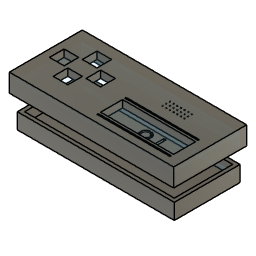
HardwareExam_LaurensController (Autodesk Fusion 360 design; units mm, degrees)
Autodesk Fusion 360 part; units mm, degrees
sketch "Sketch1" plane through (0, 0, 0) normal (0, 0, 1) x (1, 0, 0)
  line L0 (0, 110) -> (450, 110)
  line L1 (450, 110) -> (450, -90)
  line L2 (450, -90) -> (0, -90)
  line L3 (0, -90) -> (0, 110)
  dimension "d1" = 450
  dimension "d2" = 200
  constraint horizontal L0
  constraint vertical L1
  constraint horizontal L2
  constraint vertical L3
  measures "d1" distance of L0.start L0.end
  measures "d2" distance of L0.start L2.end
extrude "Extrude1" add sketch "Sketch1" against normal blind 30 makes body 1
sketch "Sketch2" plane through (0, 0, 0) normal (0, 0, 1) x (-1, 0, 0)
  line L0 (0, 90) -> (-450, 90)
  line L1 (-450, 90) -> (-450, -110)
  line L2 (-450, -110) -> (0, -110)
  line L3 (0, -110) -> (0, 90)
  line L4 (-220, 0) -> (-420, 0)
  line L5 (-420, 0) -> (-420, 60)
  line L6 (-420, 60) -> (-220, 60)
  line L7 (-220, 60) -> (-220, 0)
  line L8 (-70, -80) -> (-110, -80)
  line L9 (-110, -80) -> (-110, -40)
  line L10 (-110, -40) -> (-70, -40)
  line L11 (-70, -40) -> (-70, -80)
  line L12 (-110, 0) -> (-110, 40)
  line L13 (-70, 0) -> (-110, 0)
  line L14 (-70, 40) -> (-70, 0)
  line L15 (-110, 40) -> (-70, 40)
  line L16 (-160, -40) -> (-160, 0)
  line L17 (-120, -40) -> (-160, -40)
  line L18 (-120, 0) -> (-120, -40)
  line L19 (-160, 0) -> (-120, 0)
  line L20 (-60, -40) -> (-60, 0)
  line L21 (-20, -40) -> (-60, -40)
  line L22 (-20, 0) -> (-20, -40)
  line L23 (-60, 0) -> (-20, 0)
  dimension "d5" = 200
  dimension "d6" = 40
  dimension "d7" = 40
  dimension "d8" = 40
  dimension "d9" = 40
  dimension "d10" = 40
  dimension "d11" = 40
  dimension "d12" = 40
  dimension "d13" = 40
  constraint horizontal L4
  constraint vertical L5
  constraint horizontal L6
  constraint vertical L7
  constraint horizontal L8
  constraint vertical L9
  constraint horizontal L10
  constraint vertical L11
  constraint horizontal L13
  constraint vertical L12
  constraint horizontal L15
  constraint vertical L14
  constraint horizontal L17
  constraint vertical L16
  constraint horizontal L19
  constraint vertical L18
  constraint horizontal L21
  constraint vertical L20
  constraint horizontal L23
  constraint vertical L22
  measures "d5" distance of L4.start L4.end
  measures "d6" distance of L8.start L8.end
  measures "d7" distance of L8.start L10.end
  measures "d8" distance of L12.start L13.start
  measures "d9" distance of L14.start L13.start
  measures "d10" distance of L16.start L17.start
  measures "d11" distance of L18.start L17.start
  measures "d12" distance of L20.start L21.start
  measures "d13" distance of L22.start L21.start
extrude "Extrude2" add sketch "Sketch2" along normal blind 10 contours L4 L5 L6 L7 | L8 L9 L10 L11 | L12 L13 L14 L15 | L16 L17 L18 L19 | L20 L21 L22 L23 bodies 1
sketch "Sketch3" plane through (0, 0, 0) normal (0, 0, 1) x (-1, 0, 0)
  line L0 (-70, -40) -> (-70, -80)
  line L1 (-70, -80) -> (-110, -80)
  line L2 (-110, -80) -> (-110, -40)
  line L3 (-110, -40) -> (-70, -40)
  line L4 (-220, 60) -> (-220, 0)
  line L5 (-220, 0) -> (-420, 0)
  line L6 (-420, 0) -> (-420, 60)
  line L7 (-420, 60) -> (-220, 60)
  line L8 (-60, 0) -> (-20, 0)
  line L9 (-20, 0) -> (-20, -40)
  line L10 (-20, -40) -> (-60, -40)
  line L11 (-60, -40) -> (-60, 0)
  line L12 (-160, 0) -> (-120, 0)
  line L13 (-120, 0) -> (-120, -40)
  line L14 (-120, -40) -> (-160, -40)
  line L15 (-160, -40) -> (-160, 0)
  line L16 (-110, 40) -> (-70, 40)
  line L17 (-70, 40) -> (-70, 0)
  line L18 (-70, 0) -> (-110, 0)
  line L19 (-110, 0) -> (-110, 40)
  line L20 (0, 90) -> (-450, 90)
  line L21 (-450, 90) -> (-450, -110)
  line L22 (-450, -110) -> (0, -110)
  line L23 (0, -110) -> (0, 90)
  circle A0 centre (-290, -50) radius 1.5
  circle A1 centre (-300, -50) radius 1.5
  circle A2 centre (-310, -50) radius 1.5
  circle A3 centre (-320, -50) radius 1.5
  circle A4 centre (-330, -50) radius 1.5
  circle A5 centre (-340, -50) radius 1.5
  circle A6 centre (-350, -50) radius 1.5
  dimension "d16" = 3
  dimension "d17" = 3
  dimension "d18" = 3
  dimension "d19" = 3
  dimension "d20" = 3
  dimension "d21" = 3
  dimension "d22" = 3
  measures "d16" diameter of A0
  measures "d17" diameter of A1
  measures "d18" diameter of A2
  measures "d19" diameter of A3
  measures "d20" diameter of A4
  measures "d21" diameter of A5
  measures "d22" diameter of A6
sketch "Sketch4" plane through (0, 0, 0) normal (0, 0, 1) x (-1, 0, 0)
sketch "Sketch5" plane through (0, 0, 0) normal (0, 0, 1) x (-1, 0, 0)
  circle A0 centre (-290, -60) radius 1.5
  circle A1 centre (-300, -60) radius 1.5
  circle A2 centre (-310, -60) radius 1.5
  circle A3 centre (-320, -60) radius 1.5
  circle A4 centre (-330, -60) radius 1.5
  circle A5 centre (-340, -60) radius 1.5
  circle A6 centre (-350, -60) radius 1.5
  circle A7 centre (-290, -40) radius 1.5
  circle A8 centre (-300, -40) radius 1.5
  circle A9 centre (-310, -40) radius 1.5
  circle A10 centre (-320, -40) radius 1.5
  circle A11 centre (-330, -40) radius 1.5
  circle A12 centre (-340, -40) radius 1.5
  circle A13 centre (-350, -40) radius 1.5
  dimension "d23" = 3
  dimension "d24" = 3
  dimension "d25" = 3
  dimension "d26" = 3
  dimension "d27" = 3
  dimension "d28" = 3
  dimension "d29" = 3
  dimension "d30" = 3
  dimension "d31" = 3
  dimension "d32" = 3
  dimension "d33" = 3
  dimension "d34" = 3
  dimension "d35" = 3
  dimension "d36" = 3
  measures "d23" diameter of A0
  measures "d24" diameter of A1
  measures "d25" diameter of A2
  measures "d26" diameter of A3
  measures "d27" diameter of A4
  measures "d28" diameter of A5
  measures "d29" diameter of A6
  measures "d30" diameter of A7
  measures "d31" diameter of A8
  measures "d32" diameter of A9
  measures "d33" diameter of A10
  measures "d34" diameter of A11
  measures "d35" diameter of A12
  measures "d36" diameter of A13
extrude "Extrude3" cut sketch "Sketch3" sketch "Sketch5" against normal blind 130 contours A0 | A1 | A2 | A3 | A5 | A6 of sketch 2 bodies 1
sketch "Sketch6" plane through (0, 0, 0) normal (0, 0, 1) x (-1, 0, 0)
  circle A0 centre (-330, -40) radius 1.5
  circle A1 centre (-290, -40) radius 1.5
  circle A2 centre (-320, -60) radius 1.5
  circle A3 centre (-350, -60) radius 1.5
  circle A4 centre (-310, -60) radius 1.5
  circle A5 centre (-300, -40) radius 1.5
  circle A6 centre (-340, -40) radius 1.5
  circle A7 centre (-320, -50) radius 1.5
  circle A8 centre (-290, -50) radius 1.5
  circle A9 centre (-340, -50) radius 1.5
  circle A10 centre (-310, -50) radius 1.5
  circle A11 centre (-300, -50) radius 1.5
  circle A12 centre (-350, -50) radius 1.5
  circle A13 centre (-320, -40) radius 1.5
  circle A14 centre (-290, -60) radius 1.5
  circle A15 centre (-330, -60) radius 1.5
  circle A16 centre (-340, -60) radius 1.5
  circle A17 centre (-300, -60) radius 1.5
  circle A18 centre (-310, -40) radius 1.5
  circle A19 centre (-350, -40) radius 1.5
  line L0 (-70, -40) -> (-70, -80)
  line L1 (-70, -80) -> (-110, -80)
  line L2 (-110, -80) -> (-110, -40)
  line L3 (-110, -40) -> (-70, -40)
  line L4 (-220, 60) -> (-220, 0)
  line L5 (-220, 0) -> (-420, 0)
  line L6 (-420, 0) -> (-420, 60)
  line L7 (-420, 60) -> (-220, 60)
  line L8 (-60, 0) -> (-20, 0)
  line L9 (-20, 0) -> (-20, -40)
  line L10 (-20, -40) -> (-60, -40)
  line L11 (-60, -40) -> (-60, 0)
  line L12 (-160, 0) -> (-120, 0)
  line L13 (-120, 0) -> (-120, -40)
  line L14 (-120, -40) -> (-160, -40)
  line L15 (-160, -40) -> (-160, 0)
  line L16 (-110, 40) -> (-70, 40)
  line L17 (-70, 40) -> (-70, 0)
  line L18 (-70, 0) -> (-110, 0)
  line L19 (-110, 0) -> (-110, 40)
  line L20 (0, 90) -> (-450, 90)
  line L21 (-450, 90) -> (-450, -110)
  line L22 (-450, -110) -> (0, -110)
  line L23 (0, -110) -> (0, 90)
  circle A20 centre (-330, -50) radius 1.5
  dimension "d39" = 3
  measures "d39" diameter of A20
extrude "Extrude4" cut sketch "Sketch6" against normal blind 140 contours A20 bodies 1
sketch "Sketch7" plane through (0, 0, 0) normal (0, 0, 1) x (-1, 0, 0)
  circle A0 centre (-330, -50) radius 1.5
  circle A1 centre (-330, -40) radius 1.5
  circle A2 centre (-290, -40) radius 1.5
  circle A3 centre (-320, -60) radius 1.5
  circle A4 centre (-350, -60) radius 1.5
  circle A5 centre (-310, -60) radius 1.5
  circle A6 centre (-300, -40) radius 1.5
  circle A7 centre (-340, -40) radius 1.5
  circle A8 centre (-320, -50) radius 1.5
  circle A9 centre (-290, -50) radius 1.5
  circle A10 centre (-340, -50) radius 1.5
  circle A11 centre (-310, -50) radius 1.5
  circle A12 centre (-300, -50) radius 1.5
  circle A13 centre (-350, -50) radius 1.5
  circle A14 centre (-320, -40) radius 1.5
  circle A15 centre (-290, -60) radius 1.5
  circle A16 centre (-330, -60) radius 1.5
  circle A17 centre (-340, -60) radius 1.5
  circle A18 centre (-300, -60) radius 1.5
  circle A19 centre (-310, -40) radius 1.5
  circle A20 centre (-350, -40) radius 1.5
  line L0 (-70, -40) -> (-70, -80)
  line L1 (-70, -80) -> (-110, -80)
  line L2 (-110, -80) -> (-110, -40)
  line L3 (-110, -40) -> (-70, -40)
  line L4 (-220, 60) -> (-220, 0)
  line L5 (-220, 0) -> (-420, 0)
  line L6 (-420, 0) -> (-420, 60)
  line L7 (-420, 60) -> (-220, 60)
  line L8 (-60, 0) -> (-20, 0)
  line L9 (-20, 0) -> (-20, -40)
  line L10 (-20, -40) -> (-60, -40)
  line L11 (-60, -40) -> (-60, 0)
  line L12 (-160, 0) -> (-120, 0)
  line L13 (-120, 0) -> (-120, -40)
  line L14 (-120, -40) -> (-160, -40)
  line L15 (-160, -40) -> (-160, 0)
  line L16 (-110, 40) -> (-70, 40)
  line L17 (-70, 40) -> (-70, 0)
  line L18 (-70, 0) -> (-110, 0)
  line L19 (-110, 0) -> (-110, 40)
  line L20 (0, 90) -> (-450, 90)
  line L21 (-450, 90) -> (-450, -110)
  line L22 (-450, -110) -> (0, -110)
  line L23 (0, -110) -> (0, 90)
  line L24 (-220, -10) -> (-420, -10)
  line L25 (-420, -10) -> (-420, -6.5)
  line L26 (-420, -6.5) -> (-220, -6.5)
  line L27 (-220, -6.5) -> (-220, -10)
  line L28 (-220, 70) -> (-420, 70)
  line L29 (-420, 70) -> (-420, 66.5)
  line L30 (-420, 66.5) -> (-220, 66.5)
  line L31 (-220, 66.5) -> (-220, 70)
  dimension "d42" = 200
  dimension "d43" = 3.5
  dimension "d44" = 200
  dimension "d45" = 3.5
  constraint horizontal L24
  constraint vertical L25
  constraint horizontal L26
  constraint vertical L27
  constraint horizontal L28
  constraint vertical L29
  constraint horizontal L30
  constraint vertical L31
  measures "d42" distance of L24.start L24.end
  measures "d43" distance of L24.start L26.end
  measures "d44" distance of L28.start L28.end
  measures "d45" distance of L28.start L30.end
extrude "Extrude5" cut sketch "Sketch7" against normal blind 60 contours L24 L25 L26 L27 | L28 L29 L30 L31 bodies 1
extrude "Extrude6" cut 1 faces at (353.3333, -20, 10) along direction (0, 0, -1) blind 60 on bodies 1 bodies 1
extrude "Extrude7" cut 4 faces at (146.6667, 13.3333, 10) (83.3333, 66.6667, 10) (96.6667, -26.6667, 10) (46.6667, 13.3333, 10) along direction (0, 0, -1) blind 90 on bodies 1 bodies 1
sketch "Sketch8" plane through (0, 0, 0) normal (0, 0, 1) x (-1, 0, 0)
  line L0 (-420, -10) -> (-420, -6.5)
  line L1 (-420, -6.5) -> (-220, -6.5)
  line L2 (-220, -6.5) -> (-220, -10)
  line L3 (-220, -10) -> (-420, -10)
  line L4 (-420, 70) -> (-220, 70)
  line L5 (-220, 70) -> (-220, 66.5)
  line L6 (-220, 66.5) -> (-420, 66.5)
  line L7 (-420, 66.5) -> (-420, 70)
  circle A0 centre (-330, -50) radius 1.5
  circle A1 centre (-330, -40) radius 1.5
  circle A2 centre (-290, -40) radius 1.5
  circle A3 centre (-320, -60) radius 1.5
  circle A4 centre (-350, -60) radius 1.5
  circle A5 centre (-310, -60) radius 1.5
  circle A6 centre (-300, -40) radius 1.5
  circle A7 centre (-340, -40) radius 1.5
  circle A8 centre (-320, -50) radius 1.5
  circle A9 centre (-290, -50) radius 1.5
  circle A10 centre (-340, -50) radius 1.5
  circle A11 centre (-310, -50) radius 1.5
  circle A12 centre (-300, -50) radius 1.5
  circle A13 centre (-350, -50) radius 1.5
  circle A14 centre (-320, -40) radius 1.5
  circle A15 centre (-290, -60) radius 1.5
  circle A16 centre (-330, -60) radius 1.5
  circle A17 centre (-340, -60) radius 1.5
  circle A18 centre (-300, -60) radius 1.5
  circle A19 centre (-310, -40) radius 1.5
  circle A20 centre (-350, -40) radius 1.5
  line L8 (-70, -40) -> (-70, -80)
  line L9 (-70, -80) -> (-110, -80)
  line L10 (-110, -80) -> (-110, -40)
  line L11 (-110, -40) -> (-70, -40)
  line L12 (-220, 60) -> (-220, 0)
  line L13 (-220, 0) -> (-420, 0)
  line L14 (-420, 0) -> (-420, 60)
  line L15 (-420, 60) -> (-220, 60)
  line L16 (-60, 0) -> (-20, 0)
  line L17 (-20, 0) -> (-20, -40)
  line L18 (-20, -40) -> (-60, -40)
  line L19 (-60, -40) -> (-60, 0)
  line L20 (-160, 0) -> (-120, 0)
  line L21 (-120, 0) -> (-120, -40)
  line L22 (-120, -40) -> (-160, -40)
  line L23 (-160, -40) -> (-160, 0)
  line L24 (-110, 40) -> (-70, 40)
  line L25 (-70, 40) -> (-70, 0)
  line L26 (-70, 0) -> (-110, 0)
  line L27 (-110, 0) -> (-110, 40)
  line L28 (0, 90) -> (-450, 90)
  line L29 (-450, 90) -> (-450, -110)
  line L30 (-450, -110) -> (0, -110)
  line L31 (0, -110) -> (0, 90)
  line L32 (-20, -40) -> (-60, -40)
  line L33 (-60, -40) -> (-60, 0)
  line L34 (-60, 0) -> (-20, 0)
  line L35 (-20, 0) -> (-20, -40)
  constraint horizontal L32
  constraint vertical L33
  constraint horizontal L34
  constraint vertical L35
  constraint coincident L16.start L19.end
  constraint coincident L17.end L18.start
sketch "Sketch9" plane through (0, 0, -30) normal (0, 0, -1) x (1, 0, 0)
  line L0 (110, 0) -> (70, 0)
  line L1 (70, 0) -> (70, 40)
  line L2 (70, 40) -> (110, 40)
  line L3 (110, 40) -> (110, 0)
  line L4 (160, -40) -> (120, -40)
  line L5 (120, -40) -> (120, 0)
  line L6 (120, 0) -> (160, 0)
  line L7 (160, 0) -> (160, -40)
  line L8 (110, -40) -> (110, -80)
  line L9 (110, -80) -> (70, -80)
  line L10 (70, -80) -> (70, -40)
  line L11 (70, -40) -> (110, -40)
  line L12 (60, -40) -> (20, -40)
  line L13 (20, -40) -> (20, 0)
  line L14 (20, 0) -> (60, 0)
  line L15 (60, 0) -> (60, -40)
  line L16 (420, 60) -> (420, 0)
  line L17 (420, 0) -> (220, 0)
  line L18 (220, 0) -> (220, 60)
  line L19 (220, 60) -> (420, 60)
  line L20 (420, -6.5) -> (420, -10)
  line L21 (420, -10) -> (220, -10)
  line L22 (220, -10) -> (220, -6.5)
  line L23 (220, -6.5) -> (420, -6.5)
  line L24 (220, 70) -> (420, 70)
  line L25 (420, 70) -> (420, 66.5)
  line L26 (420, 66.5) -> (220, 66.5)
  line L27 (220, 66.5) -> (220, 70)
  circle A0 centre (330, -50) radius 1.5
  circle A1 centre (330, -40) radius 1.5
  circle A2 centre (290, -40) radius 1.5
  circle A3 centre (320, -60) radius 1.5
  circle A4 centre (350, -60) radius 1.5
  circle A5 centre (310, -60) radius 1.5
  circle A6 centre (300, -40) radius 1.5
  circle A7 centre (340, -40) radius 1.5
  circle A8 centre (320, -50) radius 1.5
  circle A9 centre (290, -50) radius 1.5
  circle A10 centre (340, -50) radius 1.5
  circle A11 centre (310, -50) radius 1.5
  circle A12 centre (300, -50) radius 1.5
  circle A13 centre (350, -50) radius 1.5
  circle A14 centre (320, -40) radius 1.5
  circle A15 centre (290, -60) radius 1.5
  circle A16 centre (330, -60) radius 1.5
  circle A17 centre (340, -60) radius 1.5
  circle A18 centre (300, -60) radius 1.5
  circle A19 centre (310, -40) radius 1.5
  circle A20 centre (350, -40) radius 1.5
  line L28 (450, 90) -> (0, 90)
  line L29 (0, 90) -> (0, -110)
  line L30 (0, -110) -> (450, -110)
  line L31 (450, -110) -> (450, 90)
  line L32 (10, 80) -> (440, 80)
  line L33 (440, 80) -> (440, -100)
  line L34 (440, -100) -> (10, -100)
  line L35 (10, -100) -> (10, 80)
  dimension "d52" = 430
  dimension "d53" = 180
  dimension "d54" = 10
  dimension "d55" = 10
  constraint horizontal L32
  constraint vertical L33
  constraint horizontal L34
  constraint vertical L35
  measures "d52" distance of L32.start L32.end
  measures "d53" distance of L32.start L34.end
  measures "d54" distance of L28 L32
  measures "d55" distance of L29 L35
extrude "Extrude8" cut sketch "Sketch9" against normal blind 10 contours L32 L33 L34 L35 bodies 1
extrude "Extrude9" add 1 faces at (296.6667, -86.6667, -30) along direction (0, 0, -1) blind 20 on bodies 1 bodies 1
sketch "Sketch10" plane through (0, 0, 0) normal (0, 0, 1) x (1, 0, 0)
  line L0 (437.786, 104.0374) -> (7.786, 104.0374)
  line L1 (7.786, 104.0374) -> (7.786, -75.9626)
  line L2 (7.786, -75.9626) -> (437.786, -75.9626)
  line L3 (437.786, -75.9626) -> (437.786, 104.0374)
  dimension "d60" = 430
  dimension "d61" = 180
  constraint horizontal L0
  constraint vertical L1
  constraint horizontal L2
  constraint vertical L3
  measures "d60" distance of L0.start L0.end
  measures "d61" distance of L0.start L2.end
extrude "Extrude10" add sketch "Sketch10" against normal blind 15 separate body makes body 2
move_body "Move1" bodies 2 to x (1, 0, 0) y (0, 1, 0) z (0, 0, 1) at (0, 0, -125)
sketch "Sketch11" plane through (0, 0, -125) normal (0, 0, 1) x (-1, 0, 0)
  line L0 (-437.786, 75.9626) -> (-437.786, -104.0374)
  line L1 (-437.786, -104.0374) -> (-7.786, -104.0374)
  line L2 (-7.786, -104.0374) -> (-7.786, 75.9626)
  line L3 (-7.786, 75.9626) -> (-437.786, 75.9626)
  line L4 (-427.786, 65.9626) -> (-17.786, 65.9626)
  line L5 (-17.786, 65.9626) -> (-17.786, -94.0374)
  line L6 (-17.786, -94.0374) -> (-427.786, -94.0374)
  line L7 (-427.786, -94.0374) -> (-427.786, 65.9626)
  dimension "d64" = 410
  dimension "d65" = 160
  dimension "d66" = 10
  dimension "d67" = 10
  constraint horizontal L4
  constraint vertical L5
  constraint horizontal L6
  constraint vertical L7
  measures "d64" distance of L4.start L4.end
  measures "d65" distance of L4.start L6.end
  measures "d66" distance of L3 L4
  measures "d67" distance of L2 L5
extrude "Extrude11" add sketch "Sketch11" along normal blind 10 bodies 2
sketch "Sketch12" plane through (0, 0, -20) normal (0, 0, -1) x (1, 0, 0)
  line L0 (120, 0) -> (160, 0)
  line L1 (160, 0) -> (160, -40)
  line L2 (160, -40) -> (120, -40)
  line L3 (120, -40) -> (120, 0)
  circle A0 centre (330, -60) radius 1.5
  line L4 (220, -10) -> (220, -6.5)
  line L5 (220, -6.5) -> (420, -6.5)
  line L6 (420, -6.5) -> (420, -10)
  line L7 (420, -10) -> (220, -10)
  circle A1 centre (310, -60) radius 1.5
  circle A2 centre (290, -50) radius 1.5
  circle A3 centre (320, -60) radius 1.5
  circle A4 centre (350, -40) radius 1.5
  circle A5 centre (300, -40) radius 1.5
  circle A6 centre (340, -40) radius 1.5
  line L8 (20, 0) -> (60, 0)
  line L9 (60, 0) -> (60, -40)
  line L10 (60, -40) -> (20, -40)
  line L11 (20, -40) -> (20, 0)
  circle A7 centre (340, -60) radius 1.5
  line L12 (70, 40) -> (110, 40)
  line L13 (110, 40) -> (110, 0)
  line L14 (110, 0) -> (70, 0)
  line L15 (70, 0) -> (70, 40)
  circle A8 centre (320, -50) radius 1.5
  line L16 (420, 66.5) -> (220, 66.5)
  line L17 (220, 66.5) -> (220, 70)
  line L18 (220, 70) -> (420, 70)
  line L19 (420, 70) -> (420, 66.5)
  circle A9 centre (310, -50) radius 1.5
  circle A10 centre (350, -50) radius 1.5
  circle A11 centre (340, -50) radius 1.5
  circle A12 centre (300, -50) radius 1.5
  line L20 (220, 0) -> (220, 60)
  line L21 (220, 60) -> (420, 60)
  line L22 (420, 60) -> (420, 0)
  line L23 (420, 0) -> (220, 0)
  circle A13 centre (350, -60) radius 1.5
  line L24 (70, -80) -> (70, -40)
  line L25 (70, -40) -> (110, -40)
  line L26 (110, -40) -> (110, -80)
  line L27 (110, -80) -> (70, -80)
  circle A14 centre (330, -50) radius 1.5
  circle A15 centre (330, -40) radius 1.5
  circle A16 centre (310, -40) radius 1.5
  circle A17 centre (290, -40) radius 1.5
  circle A18 centre (300, -60) radius 1.5
  circle A19 centre (320, -40) radius 1.5
  circle A20 centre (290, -60) radius 1.5
  line L28 (10, -100) -> (440, -100)
  line L29 (440, -100) -> (440, 80)
  line L30 (440, 80) -> (10, 80)
  line L31 (10, 80) -> (10, -100)
sketch "Sketch13" plane through (440, 0, 0) normal (-1, 0, 0) x (0, -1, 0)
  line L0 (80, -50) -> (80, -20)
  line L1 (80, -20) -> (-100, -20)
  line L2 (-100, -20) -> (-100, -50)
  line L3 (-100, -50) -> (80, -50)
sketch "Sketch14" plane through (0, 0, -140) normal (0, 0, -1) x (1, 0, 0)
  line L0 (437.786, -104.0374) -> (437.786, 75.9626)
  line L1 (437.786, 75.9626) -> (7.786, 75.9626)
  line L2 (7.786, 75.9626) -> (7.786, -104.0374)
  line L3 (7.786, -104.0374) -> (437.786, -104.0374)
  line L4 (250.4045, -89.156) -> (244.4045, -89.156)
  line L5 (244.4045, -89.156) -> (244.4045, -59.156)
  line L6 (244.4045, -59.156) -> (250.4045, -59.156)
  line L7 (250.4045, -59.156) -> (250.4045, -89.156)
  line L8 (250.4045, -59.156) -> (229.8299, -59.156)
  line L9 (229.8299, -59.156) -> (229.8299, -65)
  line L10 (229.8299, -65) -> (244.4045, -65)
  circle A0 centre (210.0712, -73.24) radius 15
  circle A1 centre (210.0712, -73.24) radius 9.7915
  line L11 (212.1497, -82.8083) -> (212.1497, -88.0953)
  line L12 (207.9927, -82.8083) -> (207.9927, -88.0953)
  line L13 (207.9927, -63.6717) -> (207.9927, -58.3847)
  line L14 (212.1497, -63.6717) -> (212.1497, -58.3847)
  line L15 (200.4282, -74.9384) -> (195.1677, -74.9384)
  line L16 (200.4282, -71.5416) -> (195.1677, -71.5416)
  line L17 (219.7143, -74.9384) -> (224.9748, -74.9384)
  line L18 (219.7143, -71.5416) -> (224.9748, -71.5416)
  dimension "d70" = 6
  dimension "d71" = 30
  dimension "d72" = 30
  dimension "d73" = 55.2367
  dimension "d74" = 187.3815
  constraint horizontal L4
  constraint vertical L5
  constraint horizontal L6
  constraint vertical L7
  constraint perpendicular L5 L8
  constraint perpendicular L3 L9
  constraint coincident L5 L10.end
  constraint perpendicular L5 L10
  constraint concentric A0 A1
  constraint coincident A1 L11.start
  constraint coincident A0 L11.end
  constraint vertical L11
  constraint coincident A1 L12.start
  constraint coincident A0 L12.end
  constraint parallel L11 L12
  constraint coincident A1 L13.start
  constraint coincident A0 L13.end
  constraint parallel L12 L13
  constraint coincident A1 L14.start
  constraint coincident A0 L14.end
  constraint parallel L11 L14
  constraint coincident A1 L15.start
  constraint coincident A0 L15.end
  constraint perpendicular L13 L15
  constraint coincident A1 L16.start
  constraint coincident A0 L16.end
  constraint parallel L15 L16
  constraint coincident A1 L17.start
  constraint coincident A0 L17.end
  constraint parallel L15 L17
  constraint coincident A1 L18.start
  constraint coincident A0 L18.end
  constraint parallel L15 L18
  measures "d70" distance of L4.start L4.end
  measures "d71" distance of L4.start L6.end
  measures "d72" diameter of A0
  measures "d73" distance of L7 L15.end
  measures "d74" distance of L0 L7
extrude "Extrude12" cut sketch "Sketch14" against normal blind 60 contours L4 L5 L6 L7 L8 | L5 L8 L9 L10 | A0 A1 L14 L18 | A0 A1 L11 L17 | A0 A1 L13 L16 | A0 A1 L12 L15 bodies 2
sketch "Sketch15" plane through (0, 100, 0) normal (0, -1, 0) x (1, 0, 0)
  line L0 (440, -50) -> (440, -20)
  line L1 (440, -20) -> (10, -20)
  line L2 (10, -20) -> (10, -50)
  line L3 (10, -50) -> (440, -50)
sketch "Sketch16" plane through (0, 94.0374, 0) normal (0, -1, 0) x (1, 0, 0)
  line L0 (17.786, -125) -> (427.786, -125)
  line L1 (427.786, -125) -> (427.786, -115)
  line L2 (427.786, -115) -> (17.786, -115)
  line L3 (17.786, -115) -> (17.786, -125)
extrude "Extrude13" add 1 faces at (291.1193, 100.7041, -115) along direction (0, 0, 1) blind 18 on bodies 2 bodies 2
named bodies: "TopHalf", "BottomHalf"
